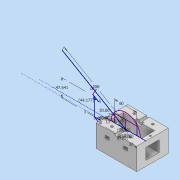
# Autodesk Inventor part: 19_Base_Pezzo_Unico
Saved by Autodesk Inventor 2020 (Build 240168000, 168)
## iProperties
Created: 2019-10-24
Part Number: 19_Base_Pezzo_Unico
Material: Generico
Document SubType Name: Modeling
Designer: socci
Density: 1 g/cm^3
Appearance: Default
Author: socci
Autodesk Inventor part; units mm, degrees
ref_plane "YZ Plane" through (0, 0, 0) normal (1, 0, 0) x (0, 1, 0)
ref_plane "XZ Plane" through (0, 0, 0) normal (0, 1, 0) x (-1, 0, 0)
ref_plane "XY Plane" through (0, 0, 0) normal (0, 0, 1) x (1, 0, 0)
sketch "Schizzo1" plane through (0, 0, 0) normal (0, 1, 0) x (-1, 0, 0)
  line L0 (55, 43) -> (-55, 43)
  line L1 (-55, 43) -> (-55, -43)
  line L2 (-55, -43) -> (55, -43)
  line L3 (55, -43) -> (55, 43)
  line L4 (55, 43) -> (-55, -43) construction
  line L5 (-55, 43) -> (55, -43) construction
  point P0 (0, 0)
  point P1 (0, 0)
  point P2 (0, 0)
  dimension "d0" = 110
  dimension "d1" = 86
  constraints: 12 end point, 3 midpoint, 2 parallel, 1 coincident, 1 horizontal, 1 perpendicular
  measures "d0" distance of L0.start L0.end
  measures "d1" distance of L2.end L0.start
extrude "Estrusione1" add sketch "Schizzo1" along normal blind 60
sketch "Schizzo2" plane through (55, 0, 43) normal (1, 0, 0) x (0, 0, -1)
  line L0 (43, 0) -> (43, 15)
  line L1 (25, 45) -> (61, 45)
  line L2 (61, 45) -> (61, 15)
  line L3 (61, 15) -> (25, 15)
  line L4 (25, 15) -> (25, 45)
  line L5 (25, 45) -> (61, 15) construction
  line L6 (61, 45) -> (25, 15) construction
  point P0 (43, 30)
  dimension "d4" = 15
  dimension "d5" = 36
  dimension "d6" = 30
  constraints: 14 end point, 3 midpoint, 2 parallel, 1 horizontal, 1 perpendicular, 1 vertical
  measures "d4" distance of L0.end L0.start
  measures "d5" distance of L1.start L1.end
  measures "d6" distance of L3.end L1.start
extrude "Estrusione2" cut sketch "Schizzo2" against normal blind 110
sketch "Schizzo3" plane through (55, 15, -18) normal (0, 0, 1) x (1, 0, 0)
  circle A0 centre (-55, 45) radius 9.5
  line L0 (0, 45) -> (-110, 45) projected
  point P0 (-55, -15)
  dimension "d9" = 19
  constraints: 1 centre point, 1 coincident, 1 midpoint
  measures "d9" diameter of A0
extrude "Estrusione3" cut sketch "Schizzo3" against normal blind 5
sketch "Schizzo4" plane through (55, 15, -23) normal (0, 0, 1) x (1, 0, 0)
  circle A0 centre (-55, 45) radius 4
  line L0 (0, 45) -> (-110, 45) projected
  point P0 (-55, -15)
  dimension "d12" = 8
  constraints: 1 centre point, 1 coincident, 1 midpoint
  measures "d12" diameter of A0
extrude "Estrusione4" cut sketch "Schizzo4" against normal blind 20
sketch "Schizzo5" plane through (55, 15, 18) normal (0, 0, -1) x (-1, 0, 0)
  circle A0 centre (55, 45) radius 9.5
  line L0 (110, 45) -> (0, 45) projected
  point P0 (55, -15)
  dimension "d15" = 19
  constraints: 1 centre point, 1 coincident, 1 midpoint
  measures "d15" diameter of A0
extrude "Estrusione5" cut sketch "Schizzo5" against normal blind 5
sketch "Schizzo6" plane through (55, 15, 23) normal (0, 0, -1) x (-1, 0, 0)
  circle A0 centre (55, 45) radius 4
  line L0 (45.5, 45) -> (64.5, 45) projected
  point P0 (55, -15)
  constraints: 1 centre point, 1 coincident, 1 midpoint
extrude "Estrusione6" cut sketch "Schizzo6" against normal blind 20
sketch "Schizzo7" plane through (0, 60, 0) normal (0, 1, 0) x (1, 0, 0)
  line L0 (-4, 43) -> (4, 43) projected
  line L1 (0, 43) -> (0, 18)
  line L2 (55, 18) -> (-55, 18) projected
  line L3 (-9.5, -18) -> (9.5, -18) projected
  line L4 (0, -18) -> (0, -43)
  line L5 (4, -43) -> (-4, -43) projected
  line L6 (-133, 18) -> (-97, 18) construction
  line L7 (-25, 30.5) -> (25, 30.5)
  line L8 (-25, -30.5) -> (25, -30.5)
  point P0 (0, 0)
  point P1 (0, 30.5)
  point P2 (0, -30.5)
  point P3 (-45, 18)
  dimension "d22" = 50
  dimension "d23" = 50
  constraints: 10 end point, 8 midpoint, 2 perpendicular, 1 horizontal
  measures "d22" distance of L7.start L7.end
  measures "d23" distance of L8.start L8.end
hole "Foro1" at (-25, 60, -30.5) at (-25, 60, 30.5) at (25, 60, 30.5) at (25, 60, -30.5) direction (0, -1, 0) diameter 5.9 depth 35 tip angle 118 clearance for "Vite a testa esagonale" size "M5" standard "ANSI - Profilo M Metrico"
sketch "Schizzo8" plane through (-55, 0, 43) normal (0, 0, 1) x (1, 0, 0)
  line L0 (27.05, 60) -> (32.95, 60) projected
  line L1 (77.05, 60) -> (82.95, 60) projected
  line L2 (80, 60) -> (80, 40)
  line L3 (80, 60) -> (60, 60) construction
  line L4 (30, 60) -> (30, 40)
  line L5 (30, 60) -> (10, 60) construction
  line L6 (25, 43.5) -> (35, 43.5)
  line L7 (35, 43.5) -> (35, 36.5)
  line L8 (35, 36.5) -> (25, 36.5)
  line L9 (25, 36.5) -> (25, 43.5)
  line L10 (25, 43.5) -> (35, 36.5) construction
  line L11 (35, 43.5) -> (25, 36.5) construction
  line L12 (75, 43.5) -> (85, 43.5)
  line L13 (85, 43.5) -> (85, 36.5)
  line L14 (85, 36.5) -> (75, 36.5)
  line L15 (75, 36.5) -> (75, 43.5)
  line L16 (75, 43.5) -> (85, 36.5) construction
  line L17 (85, 43.5) -> (75, 36.5) construction
  point P0 (55, 0)
  point P1 (30, 40)
  dimension "d31" = 90
  dimension "d32" = 270
  dimension "d33" = 20
  dimension "d34" = 20
  dimension "d35" = 7
  dimension "d36" = 7
  dimension "d37" = 10
  dimension "d38" = 10
  constraints: 32 end point, 8 midpoint, 4 horizontal, 4 parallel, 4 perpendicular
  measures "d31" angle of L2 L3
  measures "d33" distance of L4.end L4.start
  measures "d34" distance of L2.end L2.start
  measures "d35" distance of L8.end L6.start
  measures "d36" distance of L12.end L13.end
  measures "d37" distance of L7.end L8.end
  measures "d38" distance of L13.end L14.end
extrude "Estrusione7" cut sketch "Schizzo8" against normal blind 19
sketch "Schizzo10" plane through (55, 0, -43) normal (0, 0, -1) x (-1, 0, 0)
  line L0 (80, 60) -> (80, 40)
  line L1 (80, 60) -> (60, 60) construction
  line L2 (30, 60) -> (30, 40)
  line L3 (30, 60) -> (10, 60) construction
  line L4 (25, 43.5) -> (35, 43.5)
  line L5 (35, 43.5) -> (35, 36.5)
  line L6 (35, 36.5) -> (25, 36.5)
  line L7 (25, 36.5) -> (25, 43.5)
  line L8 (25, 43.5) -> (35, 36.5) construction
  line L9 (35, 43.5) -> (25, 36.5) construction
  line L10 (75, 43.5) -> (85, 43.5)
  line L11 (85, 43.5) -> (85, 36.5)
  line L12 (85, 36.5) -> (75, 36.5)
  line L13 (75, 36.5) -> (75, 43.5)
  line L14 (75, 43.5) -> (85, 36.5) construction
  line L15 (85, 43.5) -> (75, 36.5) construction
  line L16 (27.05, 60) -> (32.95, 60) projected
  line L17 (77.05, 60) -> (82.95, 60) projected
  point P0 (55, 0)
  point P1 (50, 0)
  point P2 (30, 40)
  dimension "d42" = 90
  dimension "d43" = 270
  dimension "d44" = 20
  dimension "d45" = 20
  dimension "d46" = 7
  dimension "d47" = 7
  dimension "d48" = 10
  dimension "d49" = 10
  constraints: 32 end point, 8 midpoint, 4 horizontal, 4 parallel, 4 perpendicular
  measures "d42" angle of L0 L1
  measures "d44" distance of L2.start L2.end
  measures "d45" distance of L0.start L0.end
  measures "d46" distance of L6.end L4.start
  measures "d47" distance of L10.end L11.end
  measures "d48" distance of L5.end L6.end
  measures "d49" distance of L11.end L12.end
extrude "Estrusione8" cut sketch "Schizzo10" against normal blind 19
sketch "Schizzo11" plane through (55, 15, 18) normal (0, 0, -1) x (-1, 0, 0)
  line L0 (25.0078, 67.5) -> (84.9922, 22.5) construction
  line L1 (85.0057, 68) -> (25.1859, 18.1994) construction
  line L2 (51, 45) -> (0, 45) projected
  line L3 (110, 45) -> (59, 45) projected
  line L4 (0, 45) -> (110, 45)
  line L5 (55, 45) -> (290, 45) construction
  line L6 (55, 45) -> (55, 19)
  line L7 (55, 45) -> (81, 45) construction
  line L8 (55, 19) -> (87.5948, 19) construction
  line L9 (55, 19) -> (85, 19)
  line L10 (55, 19) -> (85, 19) construction
  line L11 (55, 19) -> (25, 19)
  line L12 (27.05, 10) -> (27.05, 21.5) projected
  line L13 (55, 19) -> (85, 19) construction
  line L14 (55, 45) -> (55, 68)
  line L15 (55, 68) -> (85.0057, 68)
  line L16 (85.0057, 68) -> (25, 68)
  line L17 (25, 68) -> (25, 19)
  line L18 (25, 19) -> (85.0057, 19)
  line L19 (85.0057, 19) -> (85.0057, 68)
  circle A0 centre (55, 45) radius 39.7032
  point P0 (55, -15)
  point P1 (56.2511, 44.0615)
  dimension "d52" = 60
  dimension "d53" = 45.5
  dimension "d72" = 26
  dimension "d73" = 90
  dimension "d75" = 30
  dimension "d76" = 0
  dimension "d77" = 30
  dimension "d78" = 180
  dimension "d79" = 23
  constraints: 34 end point, 8 horizontal, 3 equal length, 3 perpendicular, 2 coincident, 2 midpoint, 2 parallel, 2 point on line, 1 collinear, 3 other
  measures "d52" distance of L0.start L1.start
  measures "d53" distance of L1.start L0.end
  measures "d72" distance of L5.start L6.end
  measures "d73" angle of L6 L7
  measures "d75" distance of L6.end L9.end
  measures "d76" distance between parallel lines of L9 L10
  measures "d77" distance of L6.end L11.end
  measures "d78" angle of L11 L13
  measures "d79" distance of L5.start L14.end
sketch "Schizzo12" plane through (55, 15, 18) normal (0, 0, -1) x (-1, 0, 0)
  line L0 (110, -15) -> (110, 45) projected
  line L1 (110, 45) -> (110, 32)
  line L2 (110, 45) -> (123, 45) construction
  line L3 (110, 32) -> (140, 32)
  line L4 (140, 32) -> (140, 35)
  line L5 (56.2511, 44.0615) -> (256.2511, 44.0615) construction
  arc A0 (51, 45) -> (59, 45) centre (55, 45) ccw projected
  line L6 (55, 45) -> (228.2051, 145)
  line L7 (55, 45) -> (255, 45) construction
  line L8 (140, 35) -> (340, 35) construction
  line L9 (145, 82.5278) -> (135, 99.8483)
  line L10 (140, 35) -> (196.188, 35) construction
  line L11 (145, 82.5278) -> (128, 72.7128)
  line L12 (140, 32) -> (140, 79.641)
  line L13 (140, 79.641) -> (140, 32)
  circle A1 centre (140, 76.1769) radius 3
  line L14 (140, 32) -> (140, 76.1769)
  line L15 (140, 32) -> (110, 10)
  point P0 (55, -15)
  point P1 (56.2511, 44.0615)
  point P2 (56.2511, 44.0615)
  dimension "d81" = 180
  dimension "d54" = 13
  dimension "d55" = 90
  dimension "d56" = 30
  dimension "d57" = 90
  dimension "d58" = 3
  dimension "d61" = 200
  dimension "d62" = 30
  dimension "d66" = 20
  dimension "d67" = 47.641
  dimension "d68" = 6
  dimension "d69" = 44.1769
  constraints: 28 end point, 4 horizontal, 3 point on line, 2 equal length, 2 perpendicular, 2 vertical, 1 centre point, 1 coincident, 1 collinear, 1 parallel, 1 tangent, 3 other
  measures "d54" distance of L0.end L1.end
  measures "d55" angle of L1 L2
  measures "d56" distance of L1.end L3.end
  measures "d57" angle of L3 L1
  measures "d58" distance of L3.end L4.end
  measures "d61" distance of L6.start L6.end
  measures "d62" angle of L7 L6
  measures "d66" distance of L9.start L9.end
  measures "d67" distance of L3.end L12.end
  measures "d68" diameter of A1
  measures "d69" distance of L3.end L14.end
sketch "Schizzo13" plane through (0, 60, 0) normal (0, 1, 0) x (1, 0, 0)
  line L0 (55, 18) -> (55, -18) projected
  line L1 (55, 18) -> (43, 18)
  line L2 (55, 18) -> (-55, 18) projected
  line L3 (55, 18) -> (67, 18) construction
  line L4 (43, 18) -> (43, -18)
  line L5 (55, -18) -> (-55, -18) projected
  line L6 (-55, -18) -> (-43, -18)
  line L7 (-43, -18) -> (-43, 18)
  line L8 (-43, 18) -> (43, 18)
  line L9 (43, 18) -> (43, -18)
  line L10 (43, -18) -> (-43, -18)
  line L11 (-43, -18) -> (-43, 18)
  line L12 (-43, 18) -> (43, 18)
  line L13 (43, 18) -> (43, -18)
  line L14 (43, -18) -> (-43, -18)
  line L15 (-43, -18) -> (-43, 18)
  point P0 (0, 0)
  point P1 (-45, 18)
  point P2 (-45, -18)
  dimension "d80" = 12
  dimension "d81" = 180
  dimension "d82" = 12
  constraints: 26 end point, 4 parallel, 4 perpendicular, 3 horizontal, 3 point on line, 2 collinear
  measures "d80" distance of L0.start L1.end
  measures "d81" angle of L1 L3
  measures "d82" distance of L5.end L6.end
extrude "Estrusione9" cut sketch "Schizzo13" against normal blind 20 contours L4 L5 L7 L2
sketch "Schizzo15" plane through (0, 60, 0) normal (0, 1, 0) x (1, 0, 0)
  line L0 (-55, 43) -> (-55, -43) projected
  line L1 (-43, -18) -> (-43, 18) projected
  line L2 (-55, 0) -> (-49, 0)
  circle A0 centre (-49, 0) radius 2.5
  line L3 (55, -43) -> (55, 43) projected
  line L4 (55, 0) -> (49, 0)
  line L5 (55, 0) -> (61, 0) construction
  circle A1 centre (49, 0) radius 2.5
  point P0 (0, 0)
  dimension "d87" = 6
  dimension "d88" = 5
  dimension "d89" = 6
  dimension "d90" = 180
  dimension "d91" = 5
  constraints: 6 end point, 3 horizontal, 2 centre point, 2 coincident, 2 midpoint, 1 collinear
  measures "d87" distance of L2.start L2.end
  measures "d88" diameter of A0
  measures "d89" distance of L4.start L4.end
  measures "d90" angle of L4 L5
  measures "d91" diameter of A1
extrude "Estrusione10" cut sketch "Schizzo15" against normal blind 15
